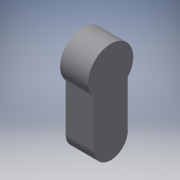
# Autodesk Inventor part: OtherCamera
Saved by Autodesk Inventor 2017 (Build 210142000, 142)
## iProperties
Created: 2017-02-18
Part Number: OtherCamera
Material: Generic
Document SubType Name: Modeling
Designer: Roksbot
Density: 1 g/cm^3
Appearance: Default
Author: Roksbot
Autodesk Inventor part; units mm, degrees
ref_plane "YZ Plane" through (0, 0, 0) normal (1, 0, 0) x (0, 1, 0)
ref_plane "XZ Plane" through (0, 0, 0) normal (0, 1, 0) x (-1, 0, 0)
ref_plane "XY Plane" through (0, 0, 0) normal (0, 0, 1) x (1, 0, 0)
sketch "Sketch1" plane through (0, 0, 0) normal (1, 0, 0) x (0, 1, 0)
  circle A0 centre (-127.5274, 0) radius 19.939
  line L0 (-73.0444, 0) -> (-182.0104, 0) construction
  line L1 (-140.6798, 14.986) -> (-182.0104, 14.986)
  line L2 (-182.0104, -14.986) -> (-140.6798, -14.986)
  arc A1 (-182.0104, 14.986) -> (-182.0104, -14.986) centre (-182.0104, 0) ccw
  point P0 (0, 0)
  dimension "d0" = 39.878
  dimension "d1" = 29.972
  dimension "d2" = 89.408
  constraints: 8 end point, 4 point on circle, 2 centre point, 2 horizontal, 2 tangent, 1 horizontal alignment, 1 midpoint, 1 parallel, 1 other
  measures "d0" diameter of A0
  measures "d1" distance between parallel lines of L1 L2
extrude "Extrusion1" add sketch "Sketch1" along normal blind 25.019
sketch "Sketch2" plane through (0, 0, 0) normal (-1, 0, 0) x (0, 0, 1)
  line L0 (0.4128, -183.6614) -> (-0.4127, -183.6614)
  line L1 (-0.4127, -183.6614) -> (-0.4127, -178.3909)
  line L2 (-0.4127, -178.3909) -> (0.4128, -178.3909)
  line L3 (0.4128, -178.3909) -> (0.4128, -183.6614)
  line L4 (0.4128, -183.6614) -> (-0.4127, -178.3909) construction
  line L5 (-0.4127, -183.6614) -> (0.4128, -178.3909) construction
  line L6 (0.4128, -152.9909) -> (-0.4127, -152.9909)
  line L7 (-0.4127, -152.9909) -> (-0.4127, -147.7204)
  line L8 (-0.4127, -147.7204) -> (0.4128, -147.7204)
  line L9 (0.4128, -147.7204) -> (0.4128, -152.9909)
  line L10 (0.4128, -152.9909) -> (-0.4127, -147.7204) construction
  line L11 (-0.4127, -152.9909) -> (0.4128, -147.7204) construction
  arc A0 (14.986, -140.6798) -> (-14.986, -140.6798) centre (0, -127.5274) ccw projected
  line L12 (-14.986, -182.0104) -> (-14.986, -140.6798) projected
  arc A1 (-14.986, -182.0104) -> (14.986, -182.0104) centre (0, -182.0104) ccw projected
  line L13 (14.986, -140.6798) -> (14.986, -182.0104) projected
  point P0 (0, 0)
  point P1 (0, -181.0262)
  point P2 (0, -150.3557)
  point P3 (0, -150.3557)
  point P4 (0, -181.0262)
  point P5 (0, -150.3557)
  dimension "d5" = 5.2705
  dimension "d6" = 0.8255
  dimension "d7" = 40.132
  dimension "d8" = 25.4
  constraints: 24 end point, 7 midpoint, 4 parallel, 2 equal length, 2 horizontal, 2 perpendicular, 2 vertical alignment, 1 point on line
  measures "d5" distance between parallel lines of L0 L2
  measures "d6" distance of L0.start L0.end
  measures "d8" distance between parallel lines of L2 L6
extrude "Extrusion2" add sketch "Sketch2" along normal blind 11.8364 contours L0 L1 L2 L3 | L6 L7 L8 L9
sketch "Sketch3" plane through (0, -183.6614, -0.4127) normal (0, 0, -1) x (-1, 0, 0)
  circle A0 centre (9.8742, 2.7496) radius 1.124
  circle A1 centre (1.6192, 2.7496) radius 1.124
  circle A2 centre (5.7086, 2.7496) radius 0.7556
  circle A3 centre (1.6192, 33.42) radius 1.124
  circle A4 centre (5.7086, 33.42) radius 0.7556
  circle A5 centre (9.8742, 33.42) radius 1.124
  line L0 (0, 0) -> (0, 5.2705) projected
  line L1 (0, 0) -> (11.8364, 0) projected
  line L2 (11.8364, 5.2705) -> (11.8364, 0) projected
  line L3 (0, 5.2705) -> (11.8364, 5.2705) projected
  line L4 (0, 30.6705) -> (0, 35.941) projected
  line L5 (0, 30.6705) -> (11.8364, 30.6705) projected
  line L6 (11.8364, 35.941) -> (11.8364, 30.6705) projected
  line L7 (0, 35.941) -> (11.8364, 35.941) projected
  point P0 (0, 183.6614)
  dimension "d11" = 2.2479
  dimension "d12" = 1.6256
  dimension "d13" = 1.6256
  dimension "d14" = 0.8382
  dimension "d15" = 1.5113
  dimension "d16" = 2.286
  dimension "d17" = 2.2479
  dimension "d18" = 2.2098
  constraints: 6 centre point, 4 horizontal alignment, 3 equal radius, 3 vertical alignment
  measures "d11" diameter of A0
  measures "d12" distance edge to line of A0 L1
  measures "d13" distance edge to line of A5 L5
  measures "d14" distance edge to line of A0 L2
  measures "d15" diameter of A2
  measures "d17" diameter of A1
extrude "Extrusion3" cut sketch "Sketch3" against normal through all contours A0 | A1 | A2 | A3 | A4 | A5
equation "\"d13\" = d12"
equation "\"d17\" = d11"
body "Solid1"
